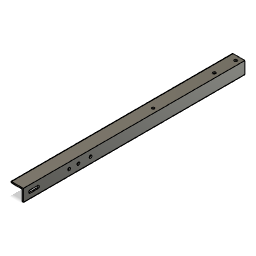
Equerre-Droite 80x80x8 longueur 1450mm (Autodesk Fusion 360 design; units mm, degrees)
Autodesk Fusion 360 part; units mm, degrees
note: some values were not read from the file. Chosen so that the rebuilt part matches the saved one: which face or edge a step refers to.
sketch "Sketch1" plane through (0, 0, 0) normal (0, 0, 1) x (1, 0, 0)
  line L0 (0, 0) -> (0, 80)
  line L1 (0, 80) -> (80, 80)
  line L2 (8, 6) -> (8, 68)
  line L3 (12, 72) -> (74, 72)
  line L4 (80, 78) -> (80, 80)
  line L5 (0, 0) -> (2, 0)
  arc A0 (74, 72) -> (80, 78) centre (74, 78) ccw
  arc A1 (2, 0) -> (8, 6) centre (2, 6) ccw
  arc A2 (12, 72) -> (8, 68) centre (12, 68) ccw
  line L6 (0, 0) -> (-2, 0)
  arc A3 (-8, 6) -> (-2, 0) centre (-2, 6) ccw
  line L7 (-8, 6) -> (-8, 68)
  arc A4 (-8, 68) -> (-12, 72) centre (-12, 68) ccw
  line L8 (-12, 72) -> (-74, 72)
  arc A5 (-80, 78) -> (-74, 72) centre (-74, 78) ccw
  line L9 (0, 80) -> (-80, 80)
  line L10 (-80, 78) -> (-80, 80)
  dimension "d1" = 80
  dimension "d2" = 80
  dimension "d4" = 6
  dimension "d5" = 6
  dimension "d6" = 4
  constraint coincident L0.start L5.start
  constraint horizontal L1
  constraint vertical L0
  constraint perpendicular L1 L4
  constraint perpendicular L2 L5
  constraint parallel L0 L2
  constraint parallel L1 L3
  constraint tangent L3 A0
  constraint tangent L4 A0
  constraint tangent L2 A1
  constraint tangent L5 A1
  constraint tangent L2 A2
  constraint tangent L3 A2
  constraint symmetric L1.start L0 L9.start
  constraint symmetric L0 L1.end L9.end
  constraint symmetric L0 L5.start L6.start
  constraint symmetric L0 L3.end L8.end
  constraint symmetric L0 L4.start A5.start
  constraint symmetric L0 A0 A5
  constraint symmetric L0 L2.start A3.start
  constraint symmetric L0 L5.end L6.end
  constraint symmetric L0 A1 A3
  constraint symmetric L0 L2.end L7.end
  constraint symmetric L0 L3.start A4.end
  constraint symmetric L0 A2 A4
  measures "d1" distance of L0.start L0.end
  measures "d2" distance of L0.end L1.end
  measures "d4" radius of A0
  measures "d5" radius of A1
  measures "d6" radius of A2
extrude "Extrude1" add sketch "Sketch1" along normal mid plane 1450
sketch "Sketch4" plane through (0, 0, 0) normal (-1, 0, 0) x (0, 0, 1)
  line L0 (-725, 0) -> (725, 0) construction
  line L1 (725, 0) -> (725, 80) construction
  line L2 (725, 80) -> (-725, 80) construction
  line L3 (-725, 80) -> (-725, 0) construction
  line L4 (-725, 0) -> (725, 0) construction
  line L5 (-725, 80) -> (725, 80) construction
  line L6 (-725, 0) -> (-725, 80) construction
  line L7 (725, 80) -> (725, 0) construction
  line L8 (0, 0) -> (0, 80) construction
  line L9 (-725, 40) -> (725, 40) construction
  line L10 (-725, 80) -> (-725, -420) construction
  line L11 (285, 80) -> (285, -420) construction
  line L12 (365, 80) -> (365, -420) construction
  line L13 (425, 80) -> (425, -420) construction
  line L14 (620, 80) -> (620, -420) construction
  line L15 (690, 80) -> (690, -420) construction
  line L16 (629, 31) -> (681, 31)
  arc A0 (681, 31) -> (681, 49) centre (681, 40) ccw
  line L17 (681, 49) -> (629, 49)
  arc A1 (629, 49) -> (629, 31) centre (629, 40) ccw
  line L18 (620, 40) -> (690, 40) construction
  circle A2 centre (285, 40) radius 9
  circle A3 centre (365, 40) radius 9
  circle A4 centre (425, 40) radius 9
  dimension "d16" = 1010
  dimension "d17" = 1090
  dimension "d18" = 1150
  dimension "d19" = 1345
  dimension "d20" = 1415
  dimension "d21" = 18
  dimension "d22" = 18
  dimension "d23" = 18
  dimension "d24" = 18
  constraint coincident L8.start origin
  constraint midpoint L2 L8.end
  constraint midpoint L3 L9.start
  constraint midpoint L7 L9.end
  constraint coincident L2.end L3.start
  constraint vertical L10
  constraint tangent L16 A0
  constraint tangent A0 L17
  constraint parallel L16 L17
  constraint tangent L17 A1
  constraint tangent L16 A1
  constraint midpoint A1 L18.start
  constraint midpoint A0 L18.end
  constraint coincident L9 L18.end
  constraint coincident L15 L18.end
  constraint perpendicular L15 L18
  constraint coincident L9 L18.start
  constraint coincident L14 L18.start
  constraint coincident L11 A2.centre
  constraint coincident L9 A2.centre
  constraint coincident L12 A3.centre
  constraint coincident L9 A3.centre
  constraint coincident L13 A4.centre
  constraint coincident L9 A4.centre
  measures "d21" diameter of A0
  measures "d22" diameter of A2
  measures "d23" diameter of A3
  measures "d24" diameter of A4
extrude "Extrude4" cut sketch "Sketch4" against normal through all and the other way through all
sketch "Sketch5" plane through (0, 80, 0) normal (0, 1, 0) x (-1, 0, 0)
  line L0 (80, 725) -> (-80, 725)
  line L1 (-80, 725) -> (-80, -725) construction
  line L2 (-80, -725) -> (80, -725) construction
  line L3 (-80, -725) -> (-80, 725) construction
  line L4 (80, -725) -> (-80, -725) construction
  line L5 (0, -725) -> (0, 725) construction
  line L6 (-30, -725) -> (-30, 725) construction
  line L7 (-80, -725) -> (384.3429, -725) construction
  line L8 (-80, -695) -> (384.3429, -695) construction
  line L9 (-80, -555) -> (384.3429, -555) construction
  line L10 (-80, -155) -> (384.3429, -155) construction
  circle A0 centre (-30, -695) radius 9
  circle A1 centre (-30, -555) radius 9
  circle A2 centre (-30, -155) radius 8
  line L11 (80, -725) -> (80, 725)
  circle A3 centre (30, -155) radius 8
  circle A4 centre (30, -555) radius 9
  circle A5 centre (30, -695) radius 9
  dimension "d27" = 30
  dimension "d28" = 170
  dimension "d29" = 570
  dimension "d30" = 18
  dimension "d31" = 18
  dimension "d32" = 16
  constraint coincident L1.end L2.start
  constraint perpendicular L3 L7
  constraint coincident L8 A0.centre
  constraint coincident L6 A0.centre
  constraint coincident L9 A1.centre
  constraint coincident L6 A1.centre
  constraint coincident L10 A2.centre
  constraint coincident L6 A2.centre
  constraint symmetric L5 A0 A5
  constraint symmetric L5 A1 A4
  constraint symmetric L5 A2 A3
  measures "d30" diameter of A0
  measures "d31" diameter of A1
  measures "d32" diameter of A2
extrude "Extrude5" cut sketch "Sketch5" against normal through all
sketch "Sketch6" plane through (0, 0, 0) normal (0, 0, 1) x (1, 0, 0)
  line L0 (-80, 80) -> (80, 80) construction
  line L1 (8, 68) -> (8, 6)
  arc A0 (2, 0) -> (8, 6) centre (2, 6) ccw
  line L2 (2, 0) -> (-2, 0) construction
  arc A1 (-8, 6) -> (-2, 0) centre (-2, 6) ccw construction
  line L3 (-8, 6) -> (-8, 68) construction
  line L4 (8, 6) -> (8, 68)
  arc A2 (-8, 68) -> (-12, 72) centre (-12, 68) ccw construction
  line L5 (-12, 72) -> (-74, 72) construction
  arc A3 (12, 72) -> (8, 68) centre (12, 68) ccw
  line L6 (74, 72) -> (12, 72)
  arc A4 (74, 72) -> (80, 78) centre (74, 78) ccw
  line L7 (80, 80) -> (80, 78)
  line L8 (-80, 78) -> (-80, 80) construction
  arc A5 (-80, 78) -> (-74, 72) centre (-74, 78) ccw construction
  line L9 (0, 80) -> (0, 0)
  line L10 (0, 80) -> (80, 80)
  line L11 (0, 0) -> (2, 0)
  constraint midpoint L0 L9.start
  constraint coincident L9.end L11.start
  constraint coincident L0.end L7.start
  constraint coincident A0.start L2.start
extrude "Extrude6" cut sketch "Sketch6" along normal mid plane 1450
